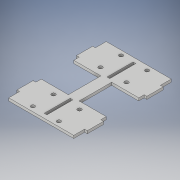
# Autodesk Inventor part: base
Saved by Autodesk Inventor 2019 (Build 230136000, 136)
## iProperties
Created: 2018-09-07
Part Number: base
Material: Generic
Document SubType Name: Modeling
Designer: mspet
Density: 1 g/cm^3
Appearance: Default
Author: mspet
Autodesk Inventor part; units mm, degrees
ref_plane "YZ Plane" through (0, 0, 0) normal (1, 0, 0) x (0, 1, 0)
ref_plane "XZ Plane" through (0, 0, 0) normal (0, 1, 0) x (-1, 0, 0)
ref_plane "XY Plane" through (0, 0, 0) normal (0, 0, 1) x (1, 0, 0)
sketch "Sketch1" plane through (0, 0, 0) normal (0, 1, 0) x (-1, 0, 0)
  line L0 (0, 0) -> (76.2, 0)
  line L1 (76.2, 0) -> (76.2, -114.3)
  line L2 (76.2, -114.3) -> (0, -114.3)
  line L3 (0, -114.3) -> (0, 0)
  dimension "d0" = 76.2
  dimension "d1" = 114.3
  constraints: 8 end point, 2 parallel, 1 horizontal, 1 perpendicular
  measures "d0" distance of L0.start L0.end
  measures "d1" distance of L2.end L0.start
extrude "Extrusion1" add sketch "Sketch1" along normal blind 3.175
sketch "Sketch2" plane through (0, 3.175, 0) normal (0, 1, 0) x (1, 0, 0)
  line L0 (0, 12.7) -> (3.175, 12.7)
  line L1 (3.175, 12.7) -> (3.175, 31.75)
  line L2 (3.175, 31.75) -> (0, 31.75)
  line L3 (0, 31.75) -> (0, 12.7)
  line L4 (0, 0) -> (0, 114.3) projected
  line L5 (0, 82.55) -> (3.175, 82.55)
  line L6 (3.175, 82.55) -> (3.175, 101.6)
  line L7 (3.175, 101.6) -> (0, 101.6)
  line L8 (0, 101.6) -> (0, 82.55)
  line L9 (-76.2, 0) -> (0, 0) projected
  line L10 (0, 114.3) -> (-76.2, 114.3) projected
  line L11 (-38.1, 0) -> (-38.1, 114.3)
  line L12 (-76.2, 12.7) -> (-79.375, 12.7)
  line L13 (-79.375, 12.7) -> (-79.375, 31.75)
  line L14 (-79.375, 31.75) -> (-76.2, 31.75)
  line L15 (-76.2, 31.75) -> (-76.2, 12.7)
  line L16 (-76.2, 0) -> (-76.2, 114.3)
  line L17 (-76.2, 82.55) -> (-79.375, 82.55)
  line L18 (-79.375, 82.55) -> (-79.375, 101.6)
  line L19 (-79.375, 101.6) -> (-76.2, 101.6)
  line L20 (-76.2, 101.6) -> (-76.2, 82.55)
  dimension "d4" = 19.05
  dimension "d5" = 19.05
  dimension "d6" = 12.7
  dimension "d7" = 12.7
  dimension "d8" = 3.175
  dimension "d9" = 3.175
  dimension "d10" = 0
  constraints: 36 end point, 8 symmetric about line, 4 parallel, 2 horizontal, 2 midpoint, 2 perpendicular, 2 point on line
  measures "d4" distance of L5.end L6.end
  measures "d5" distance of L0.end L1.end
  measures "d6" distance between parallel lines of L9 L0
  measures "d7" distance between parallel lines of L10 L7
  measures "d8" distance of L6.end L7.end
  measures "d9" distance of L0.start L0.end
  measures "d10" distance between parallel lines of L4 L3
extrude "Extrusion2" add sketch "Sketch2" against normal blind 3.175 contours L3 L2 L1 L0 | L4 L7 L6 L5 | L12 L13 L14 L15 | L16 L17 L18 L19
sketch "Sketch3" plane through (0, 3.175, 0) normal (0, 1, 0) x (1, 0, 0)
  line L0 (0, 82.55) -> (0, 31.75) projected
  line L1 (0, 38.1) -> (-31.75, 38.1)
  line L2 (-31.75, 38.1) -> (-31.75, 76.2)
  line L3 (-31.75, 76.2) -> (0, 76.2)
  line L4 (0, 76.2) -> (0, 38.1)
  line L5 (0, 82.55) -> (3.175, 82.55) projected
  line L6 (3.175, 31.75) -> (0, 31.75) projected
  line L7 (-76.2, 0) -> (0, 0) projected
  line L8 (-38.1, 0) -> (-38.1, 114.3) construction
  line L9 (0, 114.3) -> (-76.2, 114.3) projected
  line L10 (-76.2, 82.55) -> (-76.2, 31.75)
  line L11 (-76.2, 38.1) -> (-44.45, 38.1)
  line L12 (-44.45, 38.1) -> (-44.45, 76.2)
  line L13 (-44.45, 76.2) -> (-76.2, 76.2)
  line L14 (-76.2, 76.2) -> (-76.2, 38.1)
  line L15 (-76.2, 82.55) -> (-79.375, 82.55)
  line L16 (-79.375, 31.75) -> (-76.2, 31.75)
  dimension "d13" = 6.35
  dimension "d14" = 6.35
  dimension "d15" = 31.75
  constraints: 24 end point, 8 symmetric about line, 2 midpoint, 2 parallel, 2 point on line, 1 horizontal, 1 perpendicular
  measures "d13" distance between parallel lines of L3 L5
  measures "d14" distance between parallel lines of L6 L1
  measures "d15" distance between parallel lines of L0 L2
extrude "Extrusion3" cut sketch "Sketch3" against normal blind 3.175
sketch "Sketch4" plane through (0, 3.175, 0) normal (0, 1, 0) x (1, 0, 0)
  circle A0 centre (-22.86, 84.68) radius 2.2225
  circle A1 centre (-22.86, 108.81) radius 2.2225
  circle A2 centre (-53.34, 108.81) radius 2.2225
  line L0 (-31.75, 57.15) -> (-44.45, 57.15) construction
  line L1 (0, 101.6) -> (0, 114.3) projected
  circle A3 centre (-53.34, 84.68) radius 2.2225
  circle A4 centre (-22.86, 29.62) radius 2.2225
  circle A5 centre (-22.86, 5.49) radius 2.2225
  circle A6 centre (-53.34, 5.49) radius 2.2225
  circle A7 centre (-53.34, 29.62) radius 2.2225
  point P0 (0, 0)
  dimension "d24" = 4.445
  dimension "d25" = 4.445
  dimension "d26" = 4.445
  dimension "d30" = 24.13
  dimension "d33" = 30.48
  dimension "d36" = 30.48
  dimension "d37" = 22.86
  dimension "d38" = 4.445
  constraints: 8 centre point, 4 symmetric about line, 2 end point, 4 other
  measures "d24" diameter of A0
  measures "d25" diameter of A2
  measures "d26" diameter of A1
  measures "d30" distance of A0.centre A1.centre
  measures "d33" distance of A1.centre A2.centre
  measures "d36" horizontal distance of A0.centre A2.centre
  measures "d37" distance from line of L1 A1.centre
  measures "d38" diameter of A3
extrude "Extrusion4" cut sketch "Sketch4" against normal blind 3.175
sketch "Sketch5" plane through (0, 3.175, 0) normal (0, 1, 0) x (1, 0, 0)
  line L0 (-36.5125, 5.08) -> (-39.6875, 5.08)
  line L1 (-39.6875, 5.08) -> (-39.6875, 35.56)
  line L2 (-39.6875, 35.56) -> (-36.5125, 35.56)
  line L3 (-36.5125, 35.56) -> (-36.5125, 5.08)
  line L4 (-36.5125, 78.74) -> (-39.6875, 78.74)
  line L5 (-39.6875, 78.74) -> (-39.6875, 109.22)
  line L6 (-39.6875, 109.22) -> (-36.5125, 109.22)
  line L7 (-36.5125, 109.22) -> (-36.5125, 78.74)
  line L8 (-76.2, 0) -> (0, 0) projected
  line L9 (0, 114.3) -> (-76.2, 114.3) projected
  line L10 (0, 101.6) -> (0, 114.3) projected
  dimension "d39" = 3.175
  dimension "d40" = 5.08
  dimension "d41" = 5.08
  dimension "d42" = 30.48
  dimension "d43" = 30.48
  dimension "d44" = 36.5125
  constraints: 16 end point, 4 parallel, 2 horizontal, 2 perpendicular, 2 point on line
  measures "d39" distance of L4.start L4.end
  measures "d40" distance between parallel lines of L8 L0
  measures "d41" distance between parallel lines of L9 L6
  measures "d42" distance of L4.end L5.end
  measures "d43" distance of L0.end L1.end
  measures "d44" distance between parallel lines of L10 L7
extrude "Extrusion5" cut sketch "Sketch5" against normal blind 3.175
body "Solid1"
